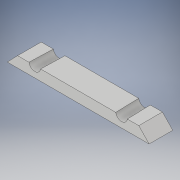
# Autodesk Inventor part: Bar_Mount_Bottom
Saved by Autodesk Inventor 2019 (Build 230136000, 136)
## iProperties
Created: 2019-08-14
Part Number: Bar_Mount_Bottom
Material: Generic
Document SubType Name: Modeling
Designer: steve
Density: 1 g/cm^3
Appearance: Default
Author: steve
Autodesk Inventor part; units mm, degrees
ref_plane "YZ Plane" through (0, 0, 0) normal (1, 0, 0) x (0, 1, 0)
ref_plane "XZ Plane" through (0, 0, 0) normal (0, 1, 0) x (-1, 0, 0)
sketch "Sketch1" plane through (0, 0, 0) normal (0, 0, 1) x (1, 0, 0)
  line L0 (90, -7.3229) -> (-90, -7.3229)
  line L1 (-90, -7.3229) -> (-76.8391, 6.2521)
  line L2 (-76.8391, 6.2521) -> (-61.4824, 6.2521)
  line L3 (76.8391, 6.2521) -> (90, -7.3229)
  line L4 (90, -7.3229) -> (-76.8391, 6.2521) construction
  line L5 (-90, -7.3229) -> (76.8391, 6.2521) construction
  line L6 (-75.8696, 7.2521) -> (77.8086, 7.2521) construction
  arc A0 (-46.7676, 6.2521) -> (-61.4824, 6.2521) centre (-54.125, 7.2521) ccw construction
  arc A1 (47.5169, 3.8663) -> (61.4824, 6.2521) centre (54.125, 7.2521) ccw
  line L7 (46.7676, 6.2521) -> (61.4824, 6.2521) construction
  line L8 (61.4824, 6.2521) -> (76.8391, 6.2521)
  arc A2 (46.7676, 6.2521) -> (47.5169, 3.8663) centre (54.125, 7.2521) ccw
  arc A3 (61.4824, 6.2521) -> (46.7676, 6.2521) centre (54.125, 7.2521) ccw construction
  line L9 (-61.4824, 6.2521) -> (-46.7676, 6.2521) construction
  line L10 (-46.7676, 6.2521) -> (46.7676, 6.2521)
  arc A4 (-47.5169, 3.8663) -> (-46.7676, 6.2521) centre (-54.125, 7.2521) ccw
  arc A5 (-61.1935, 4.9791) -> (-47.5169, 3.8663) centre (-54.125, 7.2521) ccw
  arc A6 (-61.4824, 6.2521) -> (-61.1935, 4.9791) centre (-54.125, 7.2521) ccw
  point P0 (0, 0)
  dimension "d0" = 1
  dimension "d1" = 14.85
  dimension "d2" = 54.125
  dimension "d3" = 108.25
  dimension "d5" = 180
  dimension "d6" = 22.7141
  dimension "d7" = 22.7141
  dimension "d8" = 14.575
  constraints: 22 end point, 15 point on circle, 8 point on line, 7 centre point, 6 horizontal, 5 parallel, 1 equal radius
  measures "d0" distance between parallel lines of L6 L2
  measures "d1" diameter of A0
  measures "d2" horizontal distance of point (0, 0) A0.centre
  measures "d3" distance of A1.centre A0.centre
  measures "d5" distance of L0.start L0.end
  measures "d6" horizontal distance of L1.end A0.centre
  measures "d7" horizontal distance of L3.start A1.centre
  measures "d8" distance from line of A0.centre L0
ref_plane "Work Plane1" through (0, 0, 30) normal (0, 0, 1) x (1, 0, 0)
sketch "Sketch2" plane through (0, 0, 30) normal (0, 0, 1) x (1, 0, 0)
  line L0 (90, -7.3229) -> (-90, -7.3229) projected
  line L1 (-90, -7.3229) -> (-76.8391, 6.2521) projected
  line L2 (76.8391, 6.2521) -> (90, -7.3229) projected
  line L3 (62.3824, 6.2521) -> (76.8391, 6.2521)
  line L4 (-47.6676, 6.2521) -> (47.6676, 6.2521)
  line L5 (-76.8391, 6.2521) -> (-62.3824, 6.2521)
  line L6 (-75.8696, 7.2521) -> (77.8086, 7.2521) construction
  arc A0 (-62.3824, 6.2521) -> (-47.6676, 6.2521) centre (-55.025, 7.2521) ccw
  arc A1 (47.6676, 6.2521) -> (62.3824, 6.2521) centre (55.025, 7.2521) ccw
  point P0 (0, 0)
  dimension "d10" = 7.425
  dimension "d11" = 110.05
  dimension "d12" = 55.025
  constraints: 6 end point, 4 point on circle, 2 centre point, 2 collinear, 2 point on line, 1 equal radius
  measures "d10" radius of A0
  measures "d11" distance of A1.centre A0.centre
  measures "d12" horizontal distance of A0.centre point (0, 0)
loft "Loft1" add profiles "Sketch1", "Sketch2"
equation "\"d2\" = 0.5 * d3"
equation "\"d5\" = topWidth"
equation "\"d7\" = d6"
equation "\"d10\" = 0.5 * d1"
equation "\"d12\" = 0.5 * d11"
equation "\"topWidth\" = 180"
body "Solid1"
